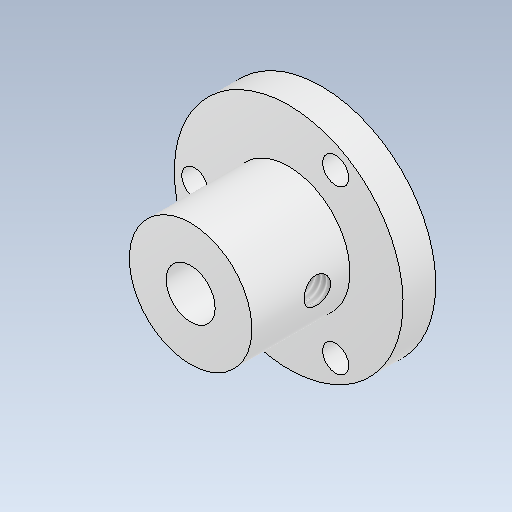
# Autodesk Inventor part: mecanum_hub
Saved by Autodesk Inventor 2026.1 (Build 301233020, 233B)
## iProperties
Created: 2026-10-09
Part Number: mecanum_hub
Material: アルミニウム 6061
Document SubType Name: Modeling
Designer: ug_nd
Density: 2.7 g/cm^3
Appearance: アルミニウム - フラット
Author: ug_nd
Autodesk Inventor part; units mm, degrees
ref_plane "YZ Plane" through (0, 0, 0) normal (1, 0, 0) x (0, 1, 0)
ref_plane "XZ Plane" through (0, 0, 0) normal (0, 1, 0) x (-1, 0, 0)
ref_plane "XY Plane" through (0, 0, 0) normal (0, 0, 1) x (1, 0, 0)
sketch "スケッチ1" plane through (0, 0, 0) normal (1, 0, 0) x (0, 1, 0)
  line L0 (0, -3.2) -> (0, 19.2) construction
  line L1 (-2.8, 0) -> (16.8, 0) construction
  line L2 (3, 16) -> (7.5, 16)
  line L3 (7.5, 16) -> (7.5, 4)
  line L4 (7.5, 4) -> (14, 4)
  line L5 (14, 4) -> (14, 0)
  line L6 (14, 0) -> (3, 0)
  line L7 (3, 0) -> (3, 16)
  point P0 (0, 0)
  dimension "d0" = 6
  dimension "d1" = 15
  dimension "d2" = 28
  dimension "d3" = 4
  dimension "d4" = 16
  constraints: 12 end point, 3 horizontal, 3 vertical, 1 point on line
  measures "d0" diameter of L7 L0
  measures "d1" diameter of L3 L0
  measures "d2" diameter of L5 L0
  measures "d3" distance between parallel lines of L1 L4
  measures "d4" distance between parallel lines of L1 L2
revolve "回転1" add sketch "スケッチ1" angle 360 about axis through (0, 0, -10) along (0, 0, 1)
sketch "スケッチ2" plane through (0, 0, 0) normal (1, 0, 0) x (0, 1, 0)
  line L0 (14, 0) -> (-14, 0) construction
  line L1 (0, -3.2) -> (0, 19.2) construction
  point P0 (0, 0)
  point P1 (0, 8)
  dimension "d8" = 8
  constraints: 1 midpoint
  measures "d8" distance from line of L0 point (0, 8)
hole "穴1" at (0, 0, 8) direction (1, 0, 0) diameter 3.242 end through all thread size "M4x0.7" class "6H" standard "ISO Metric profile"
sketch "スケッチ3" plane through (0, 0, 4) normal (0, 0, 1) x (1, 0, 0)
  circle A0 centre (-11.5, 0) radius 1.6
  line L0 (-19.6, 0) -> (19.6, 0) construction
  circle A1 centre (0, 0) radius 11.5 construction
  circle A2 centre (5.75, -9.9593) radius 1.6
  circle A3 centre (5.75, 9.9593) radius 1.6
  dimension "d16" = 23
  dimension "d17" = 3.2
  dimension "d20" = 360
  constraints: 3 centre point, 1 coincident, 1 horizontal alignment, 1 point on line, 9 other
  measures "d17" diameter of A0
extrude "押し出し1" cut sketch "スケッチ3" against normal through all
